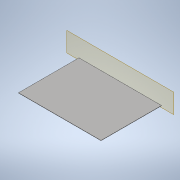
# Autodesk Inventor part: Case_Top
Saved by Autodesk Inventor 2022.2 (Build 262287010, 287A)
## iProperties
Created: 2024-11-06
Part Number: Case_Top
Material: Generisch
Document SubType Name: Modeling
Designer: ppovolni
Density: 1 g/cm^3
Appearance: Vorgabe
Author: ppovolni
Autodesk Inventor part; units mm, degrees
ref_plane "YZ Plane" through (0, 0, 0) normal (1, 0, 0) x (0, 1, 0)
ref_plane "XZ Plane" through (0, 0, 0) normal (0, 1, 0) x (-1, 0, 0)
ref_plane "XY Plane" through (0, 0, 0) normal (0, 0, 1) x (1, 0, 0)
ref_plane "Arbeitsebene1" through (0, 0, 0) normal (0, 0, 1) x (1, 0, 0)
ref_plane "Arbeitsebene2" through (-212.483, -39.158, 300) normal (0, 0, -1) x (0, 1, 0)
sketch "Skizze1" plane through (0, 0, 0) normal (0, 0, 1) x (1, 0, 0)
  line L0 (-199.983, -39.658) -> (-205.183, -39.658) construction
  line L1 (-205.183, -39.658) -> (-205.183, -41.458) construction
  line L2 (-205.183, -41.458) -> (-202.483, -41.458) construction
  arc A0 (-98.464, -8.868) -> (-101.536, -8.868) centre (-100, 0) ccw construction
  arc A1 (-98.464, -8.868) -> (-101.536, -8.868) centre (-100, -10.3) ccw construction
  arc A2 (33.362, 5.6) -> (30.9, 2.6659) centre (33.362, 3.1) ccw construction
  line L3 (33.362, 5.6) -> (56.638, 5.6) construction
  arc A3 (59.1, 2.6659) -> (56.638, 5.6) centre (56.638, 3.1) ccw construction
  line L4 (59.1, 2.6659) -> (58.0068, -3.5341) construction
  arc A4 (55.5448, -5.6) -> (58.0068, -3.5341) centre (55.5448, -3.1) ccw construction
  line L5 (55.5448, -5.6) -> (34.4552, -5.6) construction
  arc A5 (31.9932, -3.5341) -> (34.4552, -5.6) centre (34.4552, -3.1) ccw construction
  line L6 (31.9932, -3.5341) -> (30.9, 2.6659) construction
  circle A6 centre (86.48, 0) radius 1.55 construction
  circle A7 centre (184.5, -12) radius 1.55 construction
  arc A8 (90.1211, -2.9341) -> (92.5832, -5) centre (92.5832, -2.5) ccw construction
  line L7 (90.1211, -2.9341) -> (89.2395, 2.0659) construction
  arc A9 (91.7015, 5) -> (89.2395, 2.0659) centre (91.7015, 2.5) ccw construction
  line L8 (91.7015, 5) -> (128.2985, 5) construction
  arc A10 (130.7605, 2.0659) -> (128.2985, 5) centre (128.2985, 2.5) ccw construction
  line L9 (130.7605, 2.0659) -> (129.8789, -2.9341) construction
  arc A11 (127.4168, -5) -> (129.8789, -2.9341) centre (127.4168, -2.5) ccw construction
  line L10 (127.4168, -5) -> (92.5832, -5) construction
  circle A12 centre (28.34, 0) radius 1.55 construction
  circle A13 centre (-125, 17) radius 4 construction
  arc A14 (-58.464, -8.868) -> (-61.536, -8.868) centre (-60, 0) ccw construction
  arc A15 (-58.464, -8.868) -> (-61.536, -8.868) centre (-60, -10.3) ccw construction
  circle A16 centre (61.66, 0) radius 1.55 construction
  circle A17 centre (175, 0) radius 11.8 construction
  circle A18 centre (165.5, 12) radius 1.55 construction
  circle A19 centre (133.52, 0) radius 1.55 construction
  arc A20 (-18.464, -8.868) -> (-21.536, -8.868) centre (-20, 0) ccw construction
  arc A21 (-18.464, -8.868) -> (-21.536, -8.868) centre (-20, -10.3) ccw construction
  line L11 (-152.5, 0.85) -> (-152.5, -0.85) construction
  line L12 (-152.5, -0.85) -> (-151.5453, -0.85) construction
  arc A22 (-151.5453, 0.85) -> (-151.5453, -0.85) centre (-159.5, 0) ccw construction
  line L13 (-151.5453, 0.85) -> (-152.5, 0.85) construction
  line L14 (-241.3, 44.05) -> (241.3, 44.05) construction
  line L15 (-241.3, -44.05) -> (-241.3, 44.05) construction
  line L16 (241.3, -44.05) -> (-241.3, -44.05) construction
  line L17 (241.3, 44.05) -> (241.3, -44.05) construction
  circle A23 centre (208.683, 26.542) radius 1.7 construction
  circle A24 centre (-208.683, 26.542) radius 1.7 construction
  circle A25 centre (208.683, -26.542) radius 1.7 construction
  circle A26 centre (-208.683, -26.542) radius 1.7 construction
  line L18 (-231.05, -34.35) -> (-233.95, -34.35) construction
  arc A27 (-231.05, -41.85) -> (-231.05, -34.35) centre (-231.05, -38.1) ccw construction
  line L19 (-233.95, -41.85) -> (-231.05, -41.85) construction
  arc A28 (-233.95, -34.35) -> (-233.95, -41.85) centre (-233.95, -38.1) ccw construction
  line L20 (233.95, -34.35) -> (231.05, -34.35) construction
  arc A29 (233.95, -41.85) -> (233.95, -34.35) centre (233.95, -38.1) ccw construction
  line L21 (231.05, -41.85) -> (233.95, -41.85) construction
  arc A30 (231.05, -34.35) -> (231.05, -41.85) centre (231.05, -38.1) ccw construction
  line L22 (-231.05, 41.85) -> (-233.95, 41.85) construction
  arc A31 (-231.05, 34.35) -> (-231.05, 41.85) centre (-231.05, 38.1) ccw construction
  line L23 (-233.95, 34.35) -> (-231.05, 34.35) construction
  arc A32 (-233.95, 41.85) -> (-233.95, 34.35) centre (-233.95, 38.1) ccw construction
  arc A33 (233.95, 34.35) -> (233.95, 41.85) centre (233.95, 38.1) ccw construction
  line L24 (231.05, 34.35) -> (233.95, 34.35) construction
  arc A34 (231.05, 41.85) -> (231.05, 34.35) centre (231.05, 38.1) ccw construction
  line L25 (233.95, 41.85) -> (231.05, 41.85) construction
  line L26 (205.183, -39.158) -> (199.983, -39.158) construction
  line L27 (202.483, -40.958) -> (205.183, -40.958) construction
  line L28 (205.183, -40.958) -> (205.183, -39.158) construction
  line L29 (-204.683, -39.208) -> (204.683, -39.208)
  line L30 (204.683, -39.208) -> (204.683, -40.458)
  line L31 (204.683, -40.458) -> (-204.683, -40.458)
  line L32 (-204.683, -40.458) -> (-204.683, -39.208)
  point P0 (0, 0)
  point P1 (205.183, -40.058)
  point P2 (-204.683, -39.833)
extrude "Extrusion1" add sketch "Skizze1" along normal up to surface (300 mm away)
